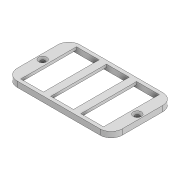
# Autodesk Inventor part: Wago2Din
Saved by Autodesk Inventor 2021 (Build 250183000, 183)
## iProperties
Created: 2021-07-31
Part Number: Wago2Din
Material: Generisch
Document SubType Name: Modeling
Designer: Rama
Density: 1 g/cm^3
Appearance: Vorgabe
Author: Rama
Autodesk Inventor part; units mm, degrees
ref_plane "YZ Plane" through (0, 0, 0) normal (1, 0, 0) x (0, 1, 0)
ref_plane "XZ Plane" through (0, 0, 0) normal (0, 1, 0) x (-1, 0, 0)
ref_plane "XY Plane" through (0, 0, 0) normal (0, 0, 1) x (1, 0, 0)
sketch "Skizze1" plane through (0, 0, 0) normal (0, 1, 0) x (-1, 0, 0)
  line L0 (28.45, 17) -> (-28.45, 17)
  line L1 (-28.45, 17) -> (-28.45, -17)
  line L2 (-28.45, -17) -> (28.45, -17)
  line L3 (28.45, -17) -> (28.45, 17)
  line L4 (28.45, 17) -> (-28.45, -17) construction
  line L5 (-28.45, 17) -> (28.45, -17) construction
  point P0 (0, 0)
  dimension "d0" = 56.9
  dimension "d1" = 34
  constraints: 12 end point, 2 midpoint, 2 parallel, 1 horizontal, 1 perpendicular
  measures "d0" distance of L2.end L1.end
  measures "d1" distance of L1.end L0.end
extrude "Extrusion1" add sketch "Skizze1" along normal blind 3
sketch "Skizze2" plane through (0, 3, 0) normal (0, 1, 0) x (1, 0, 0)
  line L0 (-6.15, -15.1) -> (6.15, -15.1)
  line L1 (6.15, -15.1) -> (6.15, 15.1)
  line L2 (6.15, 15.1) -> (-6.15, 15.1)
  line L3 (-6.15, 15.1) -> (-6.15, -15.1)
  line L4 (-6.15, -15.1) -> (6.15, 15.1) construction
  line L5 (6.15, -15.1) -> (-6.15, 15.1) construction
  line L6 (10.15, -15.1) -> (22.45, -15.1)
  line L7 (22.45, -15.1) -> (22.45, 15.1)
  line L8 (22.45, 15.1) -> (10.15, 15.1)
  line L9 (10.15, 15.1) -> (10.15, -15.1)
  line L10 (10.15, -15.1) -> (22.45, 15.1) construction
  line L11 (22.45, -15.1) -> (10.15, 15.1) construction
  line L12 (-22.45, -15.1) -> (-10.15, -15.1)
  line L13 (-10.15, -15.1) -> (-10.15, 15.1)
  line L14 (-10.15, 15.1) -> (-22.45, 15.1)
  line L15 (-22.45, 15.1) -> (-22.45, -15.1)
  line L16 (-22.45, -15.1) -> (-10.15, 15.1) construction
  line L17 (-10.15, -15.1) -> (-22.45, 15.1) construction
  line L18 (-28.45, 17) -> (-28.45, -17) projected
  line L19 (28.45, -17) -> (28.45, 17) projected
  point P0 (0, 0)
  point P1 (0, 0)
  point P2 (16.3, 0)
  point P3 (-16.3, 0)
  dimension "d4" = 12.3
  dimension "d5" = 30.2
  dimension "d6" = 12.3
  dimension "d7" = 30.2
  dimension "d8" = 12.3
  dimension "d9" = 30.2
  dimension "d10" = 4
  dimension "d11" = 4
  dimension "d12" = 6
  dimension "d13" = 6
  constraints: 36 end point, 6 midpoint, 6 parallel, 3 horizontal, 3 perpendicular, 1 coincident
  measures "d4" distance of L2.end L1.end
  measures "d5" distance of L1.end L0.end
  measures "d6" distance of L8.end L7.end
  measures "d7" distance of L7.end L6.end
  measures "d8" distance of L14.end L13.end
  measures "d9" distance of L13.end L12.end
  measures "d10" distance between parallel lines of L3 L13
  measures "d11" distance between parallel lines of L1 L9
  measures "d12" distance between parallel lines of L18 L15
  measures "d13" distance between parallel lines of L19 L7
extrude "Extrusion2" cut sketch "Skizze2" against normal blind 3
sketch "Skizze3" plane through (0, 3, 0) normal (0, 1, 0) x (1, 0, 0)
  line L0 (-25.65, 10) -> (25.65, 10)
  line L1 (25.65, 10) -> (25.65, -10)
  line L2 (25.65, -10) -> (-25.65, -10)
  line L3 (-25.65, -10) -> (-25.65, 10)
  line L4 (-25.65, 10) -> (25.65, -10) construction
  line L5 (25.65, 10) -> (-25.65, -10) construction
  line L6 (-25.65, 0) -> (25.65, 0)
  point P0 (0, 0)
  dimension "d16" = 51.3
  dimension "d17" = 20
  constraints: 14 end point, 4 midpoint, 2 parallel, 1 horizontal, 1 perpendicular
  measures "d16" distance of L1.end L2.end
  measures "d17" distance of L0.end L1.end
hole "Bohrung1" at (-25.65, 3, 0) at (25.65, 3, 0) direction (0, -1, 0) diameter 2.4 end through all countersink diameter 4.4 countersink angle 90 clearance for "Flachkopfmaschinenschraube" size "M2" standard "ANSI Metrisches M Profil"
fillet "Rundung1" radius 6 4 edges at (28.45, 1.5, 17) (28.45, 1.5, -17) (-28.45, 1.5, 17) (-28.45, 1.5, -17)
chamfer "Fase1" distance 1.5 angle 45 6 edges at (-6.15, 0, 0) (10.15, 0, 0) (6.15, 0, 0) (-10.15, 0, 0) (22.45, 0, 0) (-22.45, 0, 0)
